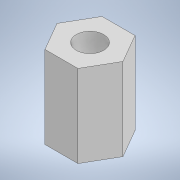
# Autodesk Inventor part: standoff
Saved by Autodesk Inventor 2022 (Build 260153000, 153)
## iProperties
Created: 2022-03-17
Part Number: standoff
Material: Generic
Document SubType Name: Modeling
Designer: 32497
Density: 1 g/cm^3
Appearance: Default
Author: 32497
Autodesk Inventor part; units mm, degrees
ref_plane "YZ Plane" through (0, 0, 0) normal (1, 0, 0) x (0, 1, 0)
ref_plane "XZ Plane" through (0, 0, 0) normal (0, 1, 0) x (-1, 0, 0)
ref_plane "XY Plane" through (0, 0, 0) normal (0, 0, 1) x (1, 0, 0)
sketch "Sketch1" plane through (0, 0, 0) normal (0, 1, 0) x (-1, 0, 0)
  circle A0 centre (0, 0) radius 1.25
  line L0 (3, 0) -> (1.5, -2.5981)
  line L1 (1.5, -2.5981) -> (-1.5, -2.5981)
  line L2 (-1.5, -2.5981) -> (-3, 0)
  line L3 (-3, 0) -> (-1.5, 2.5981)
  line L4 (-1.5, 2.5981) -> (1.5, 2.5981)
  line L5 (1.5, 2.5981) -> (3, 0)
  dimension "d0" = 2.5
  dimension "d1" = 3
  constraints: 12 end point, 2 coincident, 1 centre point, 13 other
  measures "d0" diameter of A0
  measures "d1" distance of L0.start point (0, 0)
extrude "Extrusion1" add sketch "Sketch1" along normal blind 7.5
body "Solid1"
